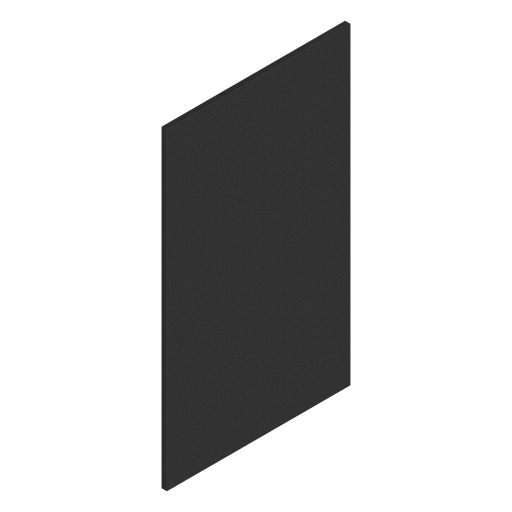
# Autodesk Inventor part: monitor
Saved by Autodesk Inventor 2023.1 (Build 271208000, 208)
## iProperties
Created: 2022-11-08
Part Number: monitor
Material: ABS Plastic
Document SubType Name: Modeling
Designer: GUT
Density: 2.04889 g/cm^3
Appearance: Black Cast
Mass: 3200 g
Surface Area: 3626.06 cm^2
Volume: 1561.82 cm^3
Author: GUT
Autodesk Inventor part; units mm, degrees
ref_plane "YZ Plane" through (0, 0, 0) normal (1, 0, 0) x (0, 1, 0)
ref_plane "XZ Plane" through (0, 0, 0) normal (0, 1, 0) x (-1, 0, 0)
ref_plane "XY Plane" through (0, 0, 0) normal (0, 0, 1) x (1, 0, 0)
sketch "Sketch1" plane through (0, 0, 0) normal (1, 0, 0) x (0, 1, 0)
  line L0 (-4.6406, 20.972) -> (539.3594, 20.972)
  line L1 (539.3594, 20.972) -> (539.3594, -298.028)
  line L2 (539.3594, -298.028) -> (-4.6406, -298.028)
  line L3 (-4.6406, -298.028) -> (-4.6406, 20.972)
  point P0 (0, 0)
  dimension "d0" = 544
  dimension "d1" = 319
  constraints: 8 end point, 2 parallel, 1 horizontal, 1 perpendicular
  measures "d0" distance of L1.end L2.end
  measures "d1" distance of L0.end L1.end
extrude "Extrusion1" add sketch "Sketch1" along normal blind 9
body "Solid1"
